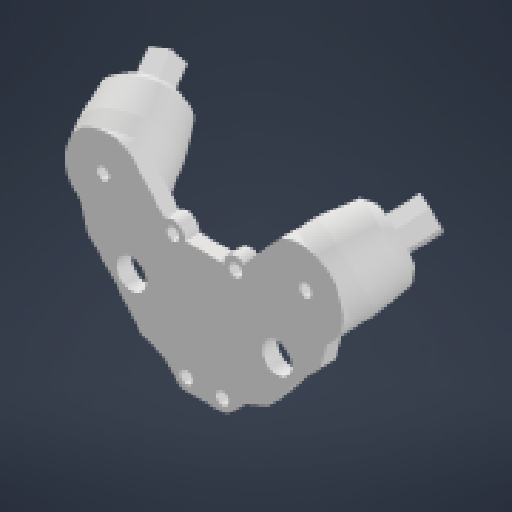
# Autodesk Inventor part: Head_Baseplate
Saved by Autodesk Inventor 2024 (Build 280153000, 153)
## iProperties
Created: 2025-09-13
Part Number: Head_Baseplate
Material: Generic
Document SubType Name: Modeling
Designer: kevin
Density: 1 g/cm^3
Appearance: Default
Author: kevin
Autodesk Inventor part; units mm, degrees
ref_plane "YZ Plane" through (0, 0, 0) normal (1, 0, 0) x (0, 1, 0)
ref_plane "XZ Plane" through (0, 0, 0) normal (0, 1, 0) x (-1, 0, 0)
sketch "Sketch1" plane through (0, 0, 0) normal (0, 0, 1) x (1, 0, 0)
  line L0 (-6.0622, -7.1524) -> (-3.0311, -1.9024) projected
  line L1 (-3.0311, -1.9024) -> (3.0311, -1.9024) projected
  line L2 (3.0311, -1.9024) -> (6.0622, -7.1524) projected
  line L3 (6.0622, -7.1524) -> (3.0311, -12.4024) projected
  line L4 (3.0311, -12.4024) -> (-3.0311, -12.4024) projected
  line L5 (-3.0311, -12.4024) -> (-6.0622, -7.1524) projected
  circle A0 centre (0, -7.1524) radius 8.6602 projected
  line L6 (0, -25.6768) -> (0, 81.9714)
  circle A1 centre (0, -7.1524) radius 13.6602
  line L7 (-5.7735, -7.1524) -> (-2.8868, -2.1524)
  line L8 (-2.8868, -2.1524) -> (2.8868, -2.1524)
  line L9 (2.8868, -2.1524) -> (5.7735, -7.1524)
  line L10 (5.7735, -7.1524) -> (2.8868, -12.1524)
  line L11 (2.8868, -12.1524) -> (-2.8868, -12.1524)
  line L12 (-2.8868, -12.1524) -> (-5.7735, -7.1524)
  point P0 (0, 0)
  point P1 (0, -12.4024)
  point P2 (0, -1.9024)
  point P3 (0, -12.1524)
  point P4 (0, -2.1524)
  dimension "d0" = 5
  dimension "d40" = 10
  constraints: 14 end point, 1 centre point, 1 coincident, 1 vertical, 13 other
  measures "d0" radial gap between concentric circles of A0 A1
  measures "d40" distance between parallel lines of L8 L11
extrude "Extrusion1" add sketch "Sketch1" against normal blind 9.85 contours L6 L11 L12 L7 L8
ref_plane "Work Plane1" through (-41.4821, 22.9354, -14.2485) normal (0.357477, -0.3940258, 0.8467313) x (-0.9336186, -0.1276658, 0.3347503)
sketch "Sketch2" plane through (-41.4821, 22.9354, -14.2485) normal (0.357477, -0.3940258, 0.8467313) x (-0.9336186, -0.1276658, 0.3347503)
  line L0 (-7.1319, -7.1524) -> (-4.1008, -1.9024) projected
  line L1 (-4.1008, -1.9024) -> (1.9614, -1.9024) projected
  line L2 (1.9614, -1.9024) -> (4.9925, -7.1524) projected
  line L3 (4.9925, -7.1524) -> (1.9614, -12.4024) projected
  line L4 (1.9614, -12.4024) -> (-4.1008, -12.4024) projected
  line L5 (-4.1008, -12.4024) -> (-7.1319, -7.1524) projected
  circle A0 centre (-1.0697, -7.1524) radius 8.6602 projected
  line L6 (4.7038, -7.1524) -> (1.8171, -12.1524)
  line L7 (1.8171, -12.1524) -> (-3.9564, -12.1524)
  line L8 (-3.9564, -12.1524) -> (-6.8432, -7.1524)
  line L9 (-6.8432, -7.1524) -> (-3.9564, -2.1524)
  line L10 (-3.9564, -2.1524) -> (1.8171, -2.1524)
  line L11 (1.8171, -2.1524) -> (4.7038, -7.1524)
  point P0 (-31.0307, 13.9963)
  dimension "d41" = 10
  constraints: 12 end point, 1 coincident, 13 other
  measures "d41" distance between parallel lines of L10 L7
extrude "Extrusion2" add sketch "Sketch2" against normal blind 11.85 contours L6 L7 L8 L9 L10 L11
sketch "Sketch3" plane through (-41.4821, 22.9354, -14.2485) normal (0.357477, -0.3940258, 0.8467313) x (0.9336186, 0.1276658, -0.3347503)
  line L0 (7.1319, 7.1524) -> (4.1008, 1.9024) projected
  line L1 (4.1008, 1.9024) -> (-1.9614, 1.9024) projected
  line L2 (-1.9614, 1.9024) -> (-4.9925, 7.1524) projected
  line L3 (-4.9925, 7.1524) -> (-1.9614, 12.4024) projected
  line L4 (-1.9614, 12.4024) -> (4.1008, 12.4024) projected
  line L5 (4.1008, 12.4024) -> (7.1319, 7.1524) projected
  circle A0 centre (1.0697, 7.1524) radius 8.6602 projected
  arc A1 (12.2217, -0.6202) -> (12.2217, 14.925) centre (1.0697, 7.1524) ccw projected
  circle A2 centre (1.0697, 7.1524) radius 13.5934
  point P0 (31.0307, -13.9963)
  point P1 (12.2217, 14.925)
  point P2 (12.2217, -0.6202)
  constraints: 1 centre point, 1 coincident
extrude "Extrusion3" add sketch "Sketch3" along normal blind 18 and the other way blind 2 contours L0 L1 L2 L3 L4 L5 | A0 | A2 A1
sketch "Sketch4" plane through (0, 0, 0) normal (0, 0, 1) x (1, 0, 0)
  line L0 (-6.0622, -7.1524) -> (-3.0311, -1.9024) projected
  line L1 (-3.0311, -1.9024) -> (3.0311, -1.9024) projected
  line L2 (3.0311, -1.9024) -> (6.0622, -7.1524) projected
  line L3 (6.0622, -7.1524) -> (3.0311, -12.4024) projected
  line L4 (3.0311, -12.4024) -> (-3.0311, -12.4024) projected
  line L5 (-3.0311, -12.4024) -> (-6.0622, -7.1524) projected
  circle A0 centre (0, -7.1524) radius 8.6602 projected
  circle A1 centre (0, -7.1524) radius 11.4859 projected
  line L6 (0, -18.6383) -> (0, 4.3335)
  point P0 (0, 0)
  constraints: 2 end point, 2 point on circle
extrude "Extrusion4" add sketch "Sketch4" along normal blind 5 contours L5 L4 L6 A0 L1 L0 | L0 L1 L6 L4 L5 | A0 L6 A1 picked at (-0.9163, -17.5851)
chamfer "Chamfer1" distance 2.9 angle 45 1 edges at (-11.4859, -7.1524, 0)
sketch "Sketch5" plane through (0, 0, 5) normal (0, 0, 1) x (1, 0, 0)
  arc A0 (0, 4.3335) -> (0, -18.6383) centre (0, -7.1524) ccw projected
  line L0 (0, -18.6383) -> (0, 4.3335) projected
  line L1 (0, 4.3335) -> (0, 53.8664)
  line L2 (-13.2174, 19.6681) -> (-23.7345, 31.5379)
  ellipse E0 centre (-33.8786, 22.4895) end of major axis (-23.811, 31.6233) minor radius 11.51 projected
  line L3 (0, -18.6383) -> (-15.5992, -18.6383) construction
  line L4 (0, -15.7383) -> (0, -18.6383) projected
  line L5 (-15.5992, -18.6383) -> (-44.0226, 13.4411)
  arc A1 (0, 4.3335) -> (0, -18.6383) centre (0, -7.1524) ccw projected
  circle A2 centre (-24.3873, -1.9711) radius 5
  circle A3 centre (-6, -22.7383) radius 2.1
  arc A4 (-6, -18.6383) -> (-6, -26.8383) centre (-6, -22.7383) ccw
  line L6 (0, -18.6383) -> (0, -26.8383)
  line L7 (-6, -26.8383) -> (0, -26.8383)
  line L8 (-8.8176, -25.7167) -> (-15.5992, -18.6383)
  circle A5 centre (-10.4984, 16.5994) radius 2.1
  arc A6 (-6.3994, 16.5123) -> (-13.2174, 19.6681) centre (-10.4984, 16.5994) ccw
  line L9 (0, 16.5123) -> (-6.3994, 16.5123)
  line L10 (-13.6831, -20.6383) -> (-21.3131, -17.5516)
  line L11 (-21.3131, -17.5516) -> (-29.7415, -7.1524)
  line L12 (-29.7415, -7.1524) -> (-27.5201, -5.1841) construction
  line L13 (-41.1956, 10.413) -> (-39.0502, 2.4669)
  line L14 (-39.0502, 2.4669) -> (-29.7415, -7.1524)
  point P0 (0, 0)
  point P1 (-41.1325, 10.1792)
  point P2 (-26.2587, -6.6077)
  point P3 (-29.2155, -3.2706)
  dimension "d15" = 10
  dimension "d16" = 4.2
  dimension "d17" = 2
  dimension "d18" = 6
  dimension "d19" = 4.2
  dimension "d20" = 2
  constraints: 26 end point, 5 centre point, 5 point on circle, 4 perpendicular, 4 point on line, 2 symmetric about line, 2 tangent, 2 vertical, 1 parallel, 5 other
  measures "d15" diameter of A2
  measures "d16" diameter of A3
  measures "d17" radial gap between concentric circles of A3 A4
  measures "d18" distance from line of A3.centre L6
  measures "d19" diameter of A5
  measures "d20" radial gap between concentric circles of A5 A6
extrude "Extrusion5" add sketch "Sketch5" along normal blind 5 contours L0 A0 | A0 L6 L7 A4 L8 L5 A2 E0 L2 A6 L9 L1 | E0 | L10 L11 L14 L13 L5 A2 L8
sketch "Sketch6" plane through (0, 0, 10) normal (0, 0, 1) x (1, 0, 0)
  line L0 (-19.8075, 9.8746) -> (-73.3288, 9.8746)
  line L1 (-73.3288, 9.8746) -> (-73.3288, 47.5031)
  line L2 (-73.3288, 47.5031) -> (-19.8075, 47.5031)
  line L3 (-19.8075, 47.5031) -> (-19.8075, 9.8746)
  point P0 (0, 0)
  constraints: 8 end point, 2 parallel, 1 horizontal, 1 perpendicular
extrude "Extrusion6" cut sketch "Sketch6" along normal blind 5
sketch "Sketch7" plane through (-35.0475, 15.8429, 0.9926) normal (0.357477, -0.3940258, 0.8467313) x (0.9336186, 0.1276658, -0.3347503)
  line L0 (9.7679, 17.5986) -> (-10.9585, 0.8198) projected
  arc A0 (-10.9585, 0.8198) -> (9.7679, 17.5986) centre (1.0697, 7.1524) ccw projected
  point P0 (31.0307, -13.9963)
extrude "Extrusion7" add sketch "Sketch7" along normal up to surface surface through (-23.2869, 4.0725, 5) normal (0, 0, 1)
chamfer "Chamfer2" distance 14.0125 angle 8 2 edges at (-53.7192, 28.6346, -8.7921) (-28.3371, 32.1055, -17.8929) measured on face at (-28.1583, 31.9084, -17.4695) measured on face at (-53.5405, 28.4376, -8.3687)
chamfer "Chamfer3" distance 2.9 angle 45 2 edges at (-51.8806, 28.886, -9.4513) (-30.1757, 31.854, -17.2337)
sketch "Sketch8" plane through (0, 0, 10) normal (0, 0, 1) x (1, 0, 0)
  ellipse E0 centre (-31.1733, 19.5076) end of major axis (-20.3862, 7.6177) minor radius 13.5934 (-36.0638, 34.277) -> (-45.3984, 25.8083) ccw projected
  ellipse E1 centre (-33.8786, 22.4895) end of major axis (-23.811, 31.6233) minor radius 11.51 (-45.3984, 25.8083) -> (-44.0226, 13.4411) ccw projected
  line L0 (-44.0226, 13.4411) -> (-41.1325, 10.1792) projected
  line L1 (-13.6831, -20.6383) -> (-8.8176, -25.7167) projected
  arc A0 (-8.8176, -25.7167) -> (-6, -26.8383) centre (-6, -22.7383) ccw projected
  line L2 (-6, -26.8383) -> (0, -26.8383) projected
  line L3 (0, -26.8383) -> (0, 16.5123) projected
  line L4 (0, 16.5123) -> (-6.3994, 16.5123) projected
  arc A1 (-6.3994, 16.5123) -> (-13.2174, 19.6681) centre (-10.4984, 16.5994) ccw projected
  line L5 (-13.2174, 19.6681) -> (-23.7345, 31.5379) projected
  ellipse E2 centre (-33.8786, 22.4895) end of major axis (-23.811, 31.6233) minor radius 11.51 (-23.7345, 31.5379) -> (-36.0638, 34.277) ccw projected
  circle A2 centre (-24.3873, -1.9711) radius 5 projected
  circle A3 centre (-6, -22.7383) radius 2.1 projected
  circle A4 centre (-10.4984, 16.5994) radius 2.1 projected
  ellipse E3 centre (-41.0281, 30.37) end of major axis (-47.4894, 24.5081) minor radius 7.387 projected
  line L6 (-23.7345, 31.5379) -> (-44.0226, 13.4411) construction
  line L7 (-33.8786, 22.4895) -> (-48.9667, 39.1203) construction
  circle A5 centre (-33.8786, 22.4895) radius 2.1
  line L8 (-41.1325, 10.1792) -> (-39.0502, 2.4669) projected
  line L9 (-39.0502, 2.4669) -> (-29.7415, -7.1524) projected
  line L10 (-29.7415, -7.1524) -> (-21.3131, -17.5516) projected
  line L11 (-21.3131, -17.5516) -> (-13.6831, -20.6383) projected
  point P0 (0, 0)
  dimension "d34" = 4.2
  constraints: 4 end point, 1 centre point, 1 coincident, 4 other
  measures "d34" diameter of A5
extrude "Extrusion8" cut sketch "Sketch8" against normal blind 7 contours A5
chamfer "Chamfer4" [suppressed]
mirror "Mirror1" about plane through (0, -2.1524, 0) normal (1, 0, 0) of "Extrusion1", "Extrusion2", "Extrusion3", "Extrusion4", "Chamfer1", "Extrusion5", "Extrusion6", "Extrusion7", "Chamfer2", "Chamfer3", "Extrusion8"
body "Solid1"
